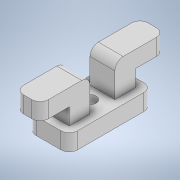
# Autodesk Inventor part: PlatformSlider
Saved by Autodesk Inventor 2022 (Build 260153000, 153)
## iProperties
Created: 2022-05-28
Part Number: PlatformSlider
Material: Generic
Document SubType Name: Modeling
Designer: victo
Density: 1 g/cm^3
Appearance: Default
Author: victo
Autodesk Inventor part; units mm, degrees
ref_plane "YZ Plane" through (0, 0, 0) normal (1, 0, 0) x (0, 1, 0)
ref_plane "XZ Plane" through (0, 0, 0) normal (0, 1, 0) x (-1, 0, 0)
ref_plane "XY Plane" through (0, 0, 0) normal (0, 0, 1) x (1, 0, 0)
sketch "Sketch1" plane through (0, 0, 0) normal (0, 1, 0) x (-1, 0, 0)
  line L0 (0, 0) -> (10, 0)
  line L1 (10, 0) -> (10, 20)
  line L2 (10, 20) -> (0, 20)
  line L3 (0, 20) -> (0, 0)
  dimension "d0" = 10
  dimension "d1" = 20
  constraints: 8 end point, 2 parallel, 1 horizontal, 1 perpendicular
  measures "d0" distance of L2.end L1.end
  measures "d1" distance of L1.end L0.end
extrude "Extrusion1" add sketch "Sketch1" along normal blind 4
sketch "Sketch2" plane through (0, 4, 0) normal (0, 1, 0) x (1, 0, 0)
  line L0 (-8, -18) -> (-2, -18)
  line L1 (-2, -18) -> (-2, -13)
  line L2 (-2, -13) -> (-8, -13)
  line L3 (-8, -13) -> (-8, -18)
  line L4 (-8, -2) -> (-2, -2)
  line L5 (-2, -2) -> (-2, -7)
  line L6 (-2, -7) -> (-8, -7)
  line L7 (-8, -7) -> (-8, -2)
  point P0 (0, 0)
  dimension "d4" = 6
  dimension "d5" = 5
  dimension "d6" = 5
  constraints: 16 end point, 4 parallel, 2 horizontal, 2 perpendicular, 2 point on line
  measures "d4" distance of L2.end L1.end
  measures "d5" distance of L1.end L0.end
  measures "d6" distance of L4.end L5.end
extrude "Extrusion2" add sketch "Sketch2" along normal blind 8
sketch "Sketch3" plane through (-8, 4, 18) normal (0, 0, 1) x (1, 0, 0)
  line L0 (0, 0) -> (0, 8) projected
  line L1 (6, 8) -> (0, 8)
  line L2 (0, 8) -> (0, 4)
  line L3 (0, 4) -> (6, 4)
  line L4 (6, 4) -> (6, 8)
  point P0 (8, -4)
  point P1 (0, 8)
  dimension "d9" = 4
  constraints: 8 end point, 2 parallel, 1 horizontal, 1 midpoint, 1 perpendicular
  measures "d9" distance of L2.end L1.end
extrude "Extrusion3" add sketch "Sketch3" along normal blind 7
sketch "Sketch4" plane through (-2, 4, 2) normal (0, 0, -1) x (-1, 0, 0)
  line L0 (0, 8) -> (6, 8) projected
  line L1 (0, 8) -> (6, 8)
  line L2 (6, 8) -> (6, 4)
  line L3 (6, 4) -> (0, 4)
  line L4 (0, 4) -> (0, 8)
  point P0 (-2, -4)
  dimension "d12" = 4
  constraints: 8 end point, 2 parallel, 1 horizontal, 1 perpendicular
  measures "d12" distance of L1.end L2.end
extrude "Extrusion4" add sketch "Sketch4" along normal blind 7
fillet "Fillet1" radius 2 8 edges at (-2, 10, -5) (-8, 10, -5) (-2, 10, 25) (-8, 10, 25) (0, 2, 20) (0, 2, 0) (-10, 2, 0) (-10, 2, 20)
sketch "Sketch5" plane through (0, 4, 0) normal (0, 1, 0) x (1, 0, 0)
  circle A0 centre (-5, -10) radius 1.5
  point P0 (0, 0)
  dimension "d16" = 3
  constraints: 1 centre point
  measures "d16" diameter of A0
extrude "Extrusion5" cut sketch "Sketch5" against normal blind 7
fillet "Fillet2" radius 2 2 edges at (-5, 12, 13) (-5, 12, 7)
body "Solid1"
